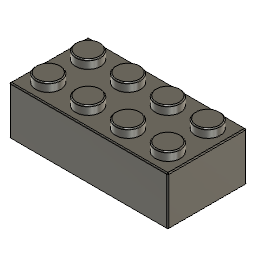
2x8 block (Autodesk Fusion 360 design; units mm, degrees)
part number: 2026-02-12-13-51-39-569
Autodesk Fusion 360 part; units mm, degrees
sketch "Sketch1" plane through (0, 0, 0) normal (0, 0, 1) x (1, 0, 0)
  line L0 (-11.8, 0) -> (20, 0)
  line L1 (20, 0) -> (20, 15.8)
  line L2 (20, 15.8) -> (-11.8, 15.8)
  line L3 (-11.8, 15.8) -> (-11.8, 0)
  dimension "d2" = 15.8
  dimension "d3" = 31.8
  constraint horizontal L0
  constraint vertical L1
  constraint horizontal L2
  constraint vertical L3
  measures "d2" distance of L0 L2
  measures "d3" distance of L1 L3
extrude "Extrude1" add sketch "Sketch1" along normal blind 9.6
sketch "Sketch2" plane through (0, 0, 9.6) normal (0, 0, 1) x (-1, 0, 0)
  line L0 (11.8, -15.8) -> (11.8, 0)
  line L1 (11.8, 0) -> (-20, 0)
  line L2 (-20, 0) -> (-20, -15.8)
  line L3 (-20, -15.8) -> (11.8, -15.8)
  circle A0 centre (-16.1, -3.9) radius 2.5
  dimension "d6" = 5
  dimension "d7" = 3.9
  dimension "d8" = 3.9
  measures "d6" diameter of A0
  measures "d7" distance of L1 A0.centre
  measures "d8" distance of L2 A0.centre
extrude "Extrude2" add sketch "Sketch2" along normal blind 1.7 contours A0
pattern_linear "R-Pattern1" count 4 spacing 8 along (-1, 0, 0) count 2 spacing 8 along (0, 1, 0) of "Extrude2"
shell "Shell1" thickness 1.49 removed faces 1 at (9.4, 10.5333, 0)
sketch "Sketch3" plane through (0, 0, 8.11) normal (0, 0, -1) x (1, 0, 0)
  circle A0 centre (-7.9, -11.9) radius 1.01
  circle A1 centre (0.1, -11.9) radius 1.01
  circle A2 centre (8.1, -11.9) radius 1.01
  circle A3 centre (16.1, -11.9) radius 1.01
  circle A4 centre (-7.9, -3.9) radius 1.01
  circle A5 centre (0.1, -3.9) radius 1.01
  circle A6 centre (8.1, -3.9) radius 1.01
  circle A7 centre (16.1, -3.9) radius 1.01
  line L0 (-10.31, -1.49) -> (-10.31, -14.31)
  line L1 (-10.31, -14.31) -> (18.51, -14.31)
  line L2 (18.51, -14.31) -> (18.51, -1.49)
  line L3 (18.51, -1.49) -> (-10.31, -1.49)
  line L4 (0.1, -3.9) -> (-7.9, -11.9) construction
  circle A8 centre (-3.9, -7.9) radius 3.15
  circle A9 centre (-3.9, -7.9) radius 2.15
  dimension "d16" = 6.3
  dimension "d18" = -1
  constraint coincident A5.centre L4.start
  constraint coincident A0.centre L4.end
  constraint midpoint L4 A8.centre
  measures "d16" diameter of A8
extrude "Extrude3" add sketch "Sketch3" along normal blind 8.1 contours A8
pattern_linear "R-Pattern2" count 1 spacing 0 along (0, 1, 0) count 3 spacing 8 along (1, 0, 0) of "Extrude3"
fillet "Fillet1" radius 0.2 16 edges at (10.4308, 4.804, 11.3) (18.4308, 4.804, 11.3) (18.4308, 12.804, 11.3) (10.4308, 12.804, 11.3) (2.4308, 12.804, 11.3) (2.4308, 4.804, 11.3) (-5.5692, 4.804, 11.3) (-5.5692, 12.804, 11.3) (-11.8, 7.9, 9.6) (4.1, 0, 9.6) (4.1, 15.8, 9.6) (20, 7.9, 9.6) (20, 15.8, 4.8) (20, 0, 4.8) (-11.8, 0, 4.8) (-11.8, 15.8, 4.8)
